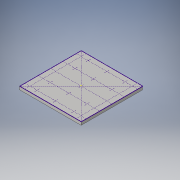
# Autodesk Inventor part: goniometer_stage_shim_v01
Saved by Autodesk Inventor 2016 (Build 200138000, 138)
## iProperties
Created: 2017-01-07
Part Number: goniometer_stage_shim_v01
Material: Generic
Document SubType Name: Modeling
Designer: stephenholtz
Density: 1 g/cm^3
Appearance: Default
Author: stephenholtz
Autodesk Inventor part; units mm, degrees
ref_plane "YZ Plane" through (0, 0, 0) normal (1, 0, 0) x (0, 1, 0)
ref_plane "XZ Plane" through (0, 0, 0) normal (0, 1, 0) x (-1, 0, 0)
ref_plane "XY Plane" through (0, 0, 0) normal (0, 0, 1) x (1, 0, 0)
sketch "adapter_holes_geom" plane through (0, 0, 0) normal (0, 0, 1) x (1, 0, 0)
  line L0 (19.05, 0) -> (-19.05, 0) construction
  line L1 (19.05, 7.62) -> (-19.05, 7.62) construction
  line L2 (19.05, -7.62) -> (-19.05, -7.62) construction
  line L3 (19.05, 19.05) -> (-19.05, 19.05)
  line L4 (-19.05, 19.05) -> (-19.05, -19.05)
  line L5 (-19.05, -19.05) -> (19.05, -19.05)
  line L6 (19.05, -19.05) -> (19.05, 19.05)
  line L7 (15.875, 19.05) -> (15.875, -19.05) construction
  line L8 (-15.875, 19.05) -> (-15.875, -19.05) construction
  line L9 (19.05, 15.875) -> (-19.05, 15.875) construction
  line L10 (19.05, -15.875) -> (-19.05, -15.875) construction
  line L11 (-19.05, 19.05) -> (19.05, 19.05) construction
  line L12 (19.05, 19.05) -> (19.05, -19.05) construction
  line L13 (19.05, -19.05) -> (-19.05, -19.05) construction
  line L14 (-19.05, -19.05) -> (-19.05, 19.05) construction
  line L15 (-19.05, 19.05) -> (19.05, -19.05) construction
  line L16 (19.05, 19.05) -> (-19.05, -19.05) construction
  point P0 (0, 0)
  point P1 (0, 0)
  point P2 (11.43, 7.62)
  point P3 (11.43, -7.62)
  point P4 (-11.43, 7.62)
  point P5 (-11.43, -7.62)
  point P6 (0, -7.62)
  point P7 (0, 7.62)
  point P8 (11.43, -15.875)
  point P9 (-11.43, -15.875)
  point P10 (0, 15.875)
  point P11 (0, -15.875)
  point P12 (0, -15.875)
  point P13 (0, 15.875)
  point P14 (11.43, 15.875)
  point P15 (-11.43, 15.875)
  dimension "d12" = 38.1
  dimension "d13" = 38.1
  dimension "d14" = 3.175
  dimension "d15" = 3.175
  dimension "d16" = 3.175
  dimension "d17" = 3.175
  dimension "d20" = 7.62
  dimension "d21" = 7.62
  dimension "d22" = 7.62
  dimension "d23" = 7.62
  dimension "d30" = 7.62
  dimension "d31" = 7.62
  dimension "d32" = 7.62
  dimension "d33" = 7.62
  dimension "d34" = 7.62
  dimension "d35" = 7.62
  measures "d12" distance of L11.end L12.end
  measures "d13" distance of L12.end L13.end
  measures "d14" distance between parallel lines of L12 L7
  measures "d15" distance between parallel lines of L11 L9
  measures "d16" distance between parallel lines of L14 L8
  measures "d17" distance between parallel lines of L13 L10
  measures "d20" distance from line of L12 point (11.43, 15.875)
  measures "d21" distance from line of L12 point (11.43, -15.875)
  measures "d22" distance from line of L14 point (-11.43, -15.875)
  measures "d23" distance from line of L14 point (-11.43, 15.875)
  measures "d30" distance between parallel lines of L0 L1
  measures "d31" distance between parallel lines of L2 L0
  measures "d32" distance from line of L6 point (11.43, 7.62)
  measures "d33" distance from line of L12 point (11.43, -7.62)
  measures "d34" distance from line of L14 point (-11.43, -7.62)
  measures "d35" distance from line of L14 point (-11.43, 7.62)
derived "goniometer_stage_top_v01.ipt"
sketch "Sketch5" plane through (0, 0, 0) normal (0, 0, 1) x (1, 0, 0)
  line L0 (19.05, 0) -> (-19.05, 0) construction
  line L1 (19.05, 7.62) -> (-19.05, 7.62) construction
  line L2 (19.05, -7.62) -> (-19.05, -7.62) construction
  line L3 (19.05, 19.05) -> (-19.05, 19.05)
  line L4 (-19.05, 19.05) -> (-19.05, -19.05)
  line L5 (-19.05, -19.05) -> (19.05, -19.05)
  line L6 (19.05, -19.05) -> (19.05, 19.05)
  line L7 (15.875, 19.05) -> (15.875, -19.05) construction
  line L8 (-15.875, 19.05) -> (-15.875, -19.05) construction
  line L9 (19.05, 15.875) -> (-19.05, 15.875) construction
  line L10 (19.05, -15.875) -> (-19.05, -15.875) construction
  line L11 (-19.05, 19.05) -> (19.05, 19.05) construction
  line L12 (19.05, 19.05) -> (19.05, -19.05) construction
  line L13 (19.05, -19.05) -> (-19.05, -19.05) construction
  line L14 (-19.05, -19.05) -> (-19.05, 19.05) construction
  line L15 (-19.05, 19.05) -> (19.05, -19.05) construction
  line L16 (19.05, 19.05) -> (-19.05, -19.05) construction
extrude "Extrusion1" add sketch "Sketch5" along normal blind 2
sketch "Sketch6" plane through (-19.05, 19.05, 2) normal (0, 0, 1) x (1, 0, 0)
  line L0 (38.1, -19.05) -> (0, -19.05) construction
  line L1 (38.1, -11.43) -> (0, -11.43) construction
  line L2 (38.1, -26.67) -> (0, -26.67) construction
  line L3 (38.1, 0) -> (0, 0)
  line L4 (0, 0) -> (0, -38.1)
  line L5 (0, -38.1) -> (38.1, -38.1)
  line L6 (38.1, -38.1) -> (38.1, 0)
  line L7 (34.925, 0) -> (34.925, -38.1) construction
  line L8 (3.175, 0) -> (3.175, -38.1) construction
  line L9 (38.1, -3.175) -> (0, -3.175) construction
  line L10 (38.1, -34.925) -> (0, -34.925) construction
  line L11 (0, 0) -> (38.1, 0) construction
  line L12 (38.1, 0) -> (38.1, -38.1) construction
  line L13 (38.1, -38.1) -> (0, -38.1) construction
  line L14 (0, -38.1) -> (0, 0) construction
  line L15 (0, 0) -> (38.1, -38.1) construction
  line L16 (38.1, 0) -> (0, -38.1) construction
  point P0 (19.05, -19.05)
  point P1 (7.62, -3.175)
  point P2 (7.62, -11.43)
  point P3 (7.62, -26.67)
  point P4 (7.62, -34.925)
  constraints: 5 other
sketch3d "adapter_holes_geom:1"
body "Solid1"
